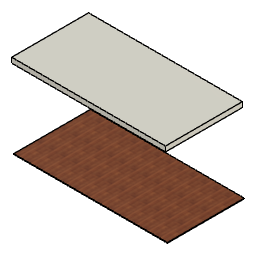
Studio (Autodesk Fusion 360 design; units mm, degrees)
Autodesk Fusion 360 part; units mm, degrees
sketch "Sketch1" plane through (0, 0, 0) normal (0, 0, 1) x (1, 0, 0) in component "Desk"
  line L0 (3000, 1500) -> (-3000, 1500)
  line L1 (-3000, 1500) -> (-3000, -1500)
  line L2 (-3000, -1500) -> (3000, -1500)
  line L3 (3000, -1500) -> (3000, 1500)
  line L4 (3000, 1500) -> (-3000, -1500) construction
  line L5 (-3000, 1500) -> (3000, -1500) construction
  dimension "d1" = 6000
  dimension "d2" = 3000
  constraint horizontal L0
  constraint perpendicular L0 L1
  constraint parallel L0 L2
  constraint parallel L1 L3
  constraint coincident L4 origin
  constraint coincident L5 origin
  measures "d1" distance of L1.end L2.end
  measures "d2" distance of L0.end L1.end
extrude "Extrude1" add sketch "Sketch1" along normal blind 20 makes body 1 in component "Desk"
ref_plane "WorkPlane1" through (0, 0, 3020) normal (0, 0, 1) x (1, 0, 0) in component "False Ceiling"
sketch "Sketch1 (2)" plane through (0, 0, 3020) normal (0, 0, 1) x (1, 0, 0) in component "False Ceiling"
  line L0 (3000, 1500) -> (-3000, 1500)
  line L1 (-3000, 1500) -> (-3000, -1500)
  line L2 (-3000, -1500) -> (3000, -1500)
  line L3 (3000, -1500) -> (3000, 1500)
  line L4 (3000, 1500) -> (-3000, -1500) construction
  line L5 (-3000, 1500) -> (3000, -1500) construction
  dimension "d12" = 6000
  dimension "d13" = 3000
  constraint horizontal L0
  constraint perpendicular L0 L1
  constraint parallel L0 L2
  constraint parallel L1 L3
  constraint coincident L4 origin
  constraint coincident L5 origin
  measures "d12" distance of L1.end L2.end
  measures "d13" distance of L0.end L1.end
extrude "Extrude1'" add sketch "Sketch1 (2)" along normal blind 200 separate body makes body 2 in component "False Ceiling"
sketch "Sketch1 (3)" plane through (0, 0, 3020) normal (0, 0, -1) x (1, 0, 0)
  line L0 (3000, -1500) -> (3000, 1500)
  line L1 (3000, 1500) -> (-3000, 1500)
  line L2 (-3000, 1500) -> (-3000, -1500)
  line L3 (-3000, -1500) -> (3000, -1500)
  line L4 (2900, 1400) -> (-2900, 1400)
  line L5 (-2900, 1400) -> (-2900, -1400)
  line L6 (-2900, -1400) -> (2900, -1400)
  line L7 (2900, -1400) -> (2900, 1400)
  line L8 (2900, 1400) -> (-2900, -1400) construction
  line L9 (-2900, 1400) -> (2900, -1400) construction
  constraint horizontal L4
  constraint perpendicular L4 L5
  constraint parallel L4 L6
  constraint parallel L5 L7
  constraint coincident L8 origin
  constraint coincident L9 origin
extrude "Extrude2" cut sketch "Sketch1 (3)" against normal blind 150 contours L4 L5 L6 L7 bodies 2 in component "False Ceiling"
sketch "Sketch1 (4)" plane through (0, 0, 3170) normal (0, 0, -1) x (1, 0, 0) in component "lights"
  line L0 (2900, -1400) -> (2900, 1400)
  line L1 (2900, 1400) -> (-2900, 1400)
  line L2 (-2900, 1400) -> (-2900, -1400)
  line L3 (-2900, -1400) -> (2900, -1400)
  circle A0 centre (-2625, 1125) radius 200
  circle A1 centre (-2625, -1125) radius 200
  circle A2 centre (2625, 1125) radius 200
  circle A3 centre (2625, -1125) radius 200
  dimension "d20" = -2250
  dimension "d21" = -5250
extrude "Extrude1''" add sketch "Sketch1 (4)" along normal blind 100 separate body contours A0 | A1 | A2 | A3 makes body 3 at (-2425.9938, 1144.9136, 3136.6667) makes body 4 at (2824.0062, -1105.0864, 3136.6667) makes body 5 at (-2425.9938, -1105.0864, 3136.6667) makes body 6 at (2824.0062, 1144.9136, 3136.6667) in component "lights"
sketch "Sketch2" plane through (0, 0, 3070) normal (0, 0, -1) x (1, 0, 0) in component "lights"
  circle A0 centre (2625, 1125) radius 200
  circle A1 centre (2625, 1125) radius 175
  circle A2 centre (2625, -1125) radius 175
  circle A3 centre (-2625, -1125) radius 175
  circle A4 centre (-2625, 1125) radius 175
  constraint concentric A0 A1
extrude "Extrude2'" cut sketch "Sketch2" against normal blind 80 contours A1 | A2 | A3 | A4 bodies 3 4 5 6 in component "lights"
component "Desk" placed x (1, 0, 0) y (0, 1, 0) z (0, 0, 1) at (152.9708, -77.3137, 54.8464)
component "False Ceiling" placed x (1, 0, 0) y (0, 1, 0) z (0, 0, 1) at (0, 0, 0)
component "lights" placed x (1, 0, 0) y (0, 1, 0) z (0, 0, 1) at (0, 0, 0)
